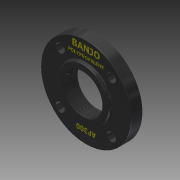
# Autodesk Inventor part: delta rythm
Saved by Autodesk Inventor 2013 SP2 (Build 170200200, 200)
## iProperties
Created: 2014-07-14
Part Number: delta rythm
Material: GFRP
Document SubType Name: Modeling
Designer: mrister
Density: 1.75 g/cm^3
Description: FLANGE, PLATIC - 3" 150#, THR'D (BANJO AF300)
Engineer: mrister
Author: mrister
Autodesk Inventor part; units mm, degrees
ref_plane "YZ Plane" through (0, 0, 0) normal (1, 0, 0) x (0, 1, 0)
ref_plane "XZ Plane" through (0, 0, 0) normal (0, 1, 0) x (-1, 0, 0)
ref_plane "XY Plane" through (0, 0, 0) normal (0, 0, 1) x (1, 0, 0)
sketch "Sketch1" plane through (0, 0, 0) normal (0, 0, 1) x (1, 0, 0)
  circle A0 centre (0, 0) radius 41.275
  circle A1 centre (0, 0) radius 95.25
  circle A2 centre (-53.8815, 53.8815) radius 9.525
  line L0 (-53.8815, 53.8815) -> (0, 0) construction
  line L1 (0, 0) -> (0, 95.25) construction
  circle A3 centre (-53.8815, -53.8815) radius 9.525
  circle A4 centre (53.8815, -53.8815) radius 9.525
  circle A5 centre (53.8815, 53.8815) radius 9.525
  dimension "d1" = 190.5
  dimension "d0" = 45
  dimension "d3" = 76.2
  dimension "d4" = 82.55
  dimension "d5" = 19.05
  dimension "d8" = 360
  constraints: 5 centre point, 4 end point, 2 coincident, 1 vertical, 1 vertical alignment, 11 other
  measures "d0" angle of L1 L0
  measures "d3" distance of L0.start L0.end
  measures "d4" diameter of A0
  measures "d5" diameter of A2
extrude "Extrusion1" add sketch "Sketch1" along normal blind 23.8125
sketch "Sketch2" plane through (0, 0, 23.8125) normal (0, 0, 1) x (1, 0, 0)
  circle A0 centre (0, 0) radius 41.275 projected
  circle A1 centre (0, 0) radius 95.25 projected
  circle A2 centre (0, 0) radius 53.975
  dimension "d12" = 107.95
  constraints: 1 centre point, 1 coincident
  measures "d12" diameter of A2
extrude "Extrusion2" add sketch "Sketch2" along normal blind 6.35 contours A2
chamfer "Chamfer1" distance 1.5875 angle 45 1 edges at (-53.975, 0, 23.8125)
fillet "Fillet1" radius 1.5875 2 edges at (-53.975, 0, 30.1625) (-95.25, 0, 23.8125)
sketch "Sketch3" plane through (0, 0, 0) normal (1, 0, 0) x (0, 1, 0)
  line L0 (41.275, 0) -> (41.275, 30.1625) projected
  line L1 (41.275, 35.0283) -> (41.275, 34.2346)
  line L2 (41.275, 34.2346) -> (42.0688, 34.6314)
  line L3 (42.0688, 34.6314) -> (41.275, 35.0283)
  line L4 (42.0688, 34.6314) -> (41.275, 34.6314) construction
  point P0 (0, 0)
  dimension "d20" = 0.7937
  constraints: 8 end point, 1 collinear, 1 horizontal, 1 midpoint, 1 perpendicular, 1 vertical
  measures "d20" distance of L1.start L1.end
coil "Coil1" sketch "Sketch3" operation cut axis through (0, 0, -10) along (0, 0, -1) pitch 0.9525 turns 160 hand right
sketch "Sketch4" plane through (0, 0, 23.8125) normal (0, 0, 1) x (1, 0, 0)
  circle A0 centre (0, 0) radius 93.6625 projected
  line L0 (-36.3748, 85.725) -> (36.3748, 85.725) construction
  line L1 (36.3748, 85.725) -> (36.3748, 60.325) construction
  line L2 (36.3748, 60.325) -> (-36.3748, 60.325) construction
  line L3 (-36.3748, 60.325) -> (-36.3748, 85.725) construction
  line L4 (0, 60.325) -> (0, 0) construction
  line L5 (12.7, -76.2) -> (-12.7, -76.2) construction
  line L6 (-12.7, -76.2) -> (-12.7, -63.5) construction
  line L7 (-12.7, -63.5) -> (12.7, -63.5) construction
  line L8 (12.7, -63.5) -> (12.7, -76.2) construction
  line L9 (0, -63.5) -> (0, 0) construction
  spline S0 degree 2 poles (-18.3296, 76.9511) (-18.3296, 76.0043) (-19.05, 74.5738) (-19.6469, 74.1003) knots 0 0 0 1 2 2 2
  spline S1 degree 2 poles (-19.6469, 74.1003) (-20.3673, 73.5343) (-22.0758, 73.0609) (-23.4034, 73.0609) knots 0 0 0 1 2 2 2
  line L10 (-23.4034, 73.0609) -> (-28.4772, 73.0609)
  line L11 (-28.4772, 73.0609) -> (-28.4772, 85.7609)
  line L12 (-28.4772, 85.7609) -> (-24.0003, 85.7609)
  spline S2 degree 2 poles (-24.0003, 85.7609) (-22.6006, 85.7609) (-21.1598, 85.5447) (-20.532, 85.2051) knots 0 0 0 1 2 2 2
  spline S3 degree 2 poles (-20.532, 85.2051) (-19.8425, 84.8449) (-19.1735, 83.6099) (-19.1735, 82.8071) knots 0 0 0 1 2 2 2
  spline S4 degree 2 poles (-19.1735, 82.8071) (-19.1735, 81.8809) (-20.0998, 80.4298) (-20.9231, 80.0901) knots 0 0 0 1 2 2 2
  line L13 (-20.9231, 80.0901) -> (-20.9231, 80.0284)
  spline S5 degree 2 poles (-20.9231, 80.0284) (-19.7395, 79.7814) (-18.3296, 78.2479) (-18.3296, 76.9511) knots 0 0 0 1 2 2 2
  spline S6 degree 2 poles (-21.6229, 77.0026) (-21.6229, 77.5995) (-22.0964, 78.2685) (-22.5698, 78.4435) knots 0 0 0 1 2 2 2
  spline S7 degree 2 poles (-22.5698, 78.4435) (-22.8579, 78.5567) (-23.8768, 78.5772) (-24.7207, 78.5772) knots 0 0 0 1 2 2 2
  line L14 (-24.7207, 78.5772) -> (-25.3074, 78.5772)
  line L15 (-25.3074, 78.5772) -> (-25.3074, 75.3765)
  line L16 (-25.3074, 75.3765) -> (-25.1324, 75.3765)
  spline S8 degree 2 poles (-25.1324, 75.3765) (-23.8974, 75.3765) (-22.9506, 75.4074) (-22.4566, 75.6235) knots 0 0 0 1 2 2 2
  spline S9 degree 2 poles (-22.4566, 75.6235) (-22.0243, 75.8191) (-21.6229, 76.5395) (-21.6229, 77.0026) knots 0 0 0 1 2 2 2
  spline S10 degree 2 poles (-22.4154, 82.1793) (-22.4154, 82.4881) (-22.7344, 83.1365) (-23.0638, 83.2806) knots 0 0 0 1 2 2 2
  spline S11 degree 2 poles (-23.0638, 83.2806) (-23.3725, 83.4246) (-24.237, 83.4452) (-25.0912, 83.4452) knots 0 0 0 1 2 2 2
  line L17 (-25.0912, 83.4452) -> (-25.3074, 83.4452)
  line L18 (-25.3074, 83.4452) -> (-25.3074, 80.7488)
  line L19 (-25.3074, 80.7488) -> (-24.906, 80.7488)
  spline S12 degree 2 poles (-24.906, 80.7488) (-24.0929, 80.7488) (-23.4343, 80.7797) (-23.0844, 80.9443) knots 0 0 0 1 2 2 2
  spline S13 degree 2 poles (-23.0844, 80.9443) (-22.7036, 81.1296) (-22.4154, 81.7574) (-22.4154, 82.1793) knots 0 0 0 1 2 2 2
  line L20 (-17.8664, 73.0609) -> (-13.5748, 85.7609)
  line L21 (-13.5748, 85.7609) -> (-10.0962, 85.7609)
  line L22 (-10.0962, 85.7609) -> (-5.8045, 73.0609)
  line L23 (-5.8045, 73.0609) -> (-9.0876, 73.0609)
  line L24 (-9.0876, 73.0609) -> (-9.8801, 75.6544)
  line L25 (-9.8801, 75.6544) -> (-13.8733, 75.6544)
  line L26 (-13.8733, 75.6544) -> (-14.676, 73.0609)
  line L27 (-14.676, 73.0609) -> (-17.8664, 73.0609)
  line L28 (-10.5799, 77.9597) -> (-11.8767, 82.1588)
  line L29 (-11.8767, 82.1588) -> (-13.1837, 77.9597)
  line L30 (-13.1837, 77.9597) -> (-10.5799, 77.9597)
  line L31 (6.3397, 73.0609) -> (3.2728, 73.0609)
  line L32 (3.2728, 73.0609) -> (-1.6261, 81.9118)
  line L33 (-1.6261, 81.9118) -> (-1.6261, 73.0609)
  line L34 (-1.6261, 73.0609) -> (-4.5387, 73.0609)
  line L35 (-4.5387, 73.0609) -> (-4.5387, 85.7609)
  line L36 (-4.5387, 85.7609) -> (-0.6278, 85.7609)
  line L37 (-0.6278, 85.7609) -> (3.4271, 78.4846)
  line L38 (3.4271, 78.4846) -> (3.4271, 85.7609)
  line L39 (3.4271, 85.7609) -> (6.3397, 85.7609)
  line L40 (6.3397, 85.7609) -> (6.3397, 73.0609)
  spline S14 degree 2 poles (15.1906, 76.7865) (15.1906, 75.9631) (14.6246, 74.5017) (14.0585, 73.9871) knots 0 0 0 1 2 2 2
  spline S15 degree 2 poles (14.0585, 73.9871) (13.4204, 73.4108) (11.6811, 72.8653) (10.549, 72.8653) knots 0 0 0 1 2 2 2
  spline S16 degree 2 poles (10.549, 72.8653) (9.7051, 72.8653) (8.2231, 72.9888) (7.6571, 73.1123) knots 0 0 0 1 2 2 2
  line L41 (7.6571, 73.1123) -> (7.6571, 75.6853)
  line L42 (7.6571, 75.6853) -> (7.9452, 75.6853)
  spline S17 degree 2 poles (7.9452, 75.6853) (8.326, 75.5309) (9.1596, 75.2633) (9.8183, 75.2633) knots 0 0 0 1 2 2 2
  spline S18 degree 2 poles (9.8183, 75.2633) (10.6622, 75.2633) (11.5782, 75.7367) (11.7635, 76.169) knots 0 0 0 1 2 2 2
  spline S19 degree 2 poles (11.7635, 76.169) (11.959, 76.5909) (12.0002, 77.6819) (12.0002, 78.3611) knots 0 0 0 1 2 2 2
  line L43 (12.0002, 78.3611) -> (12.0002, 83.4555)
  line L44 (12.0002, 83.4555) -> (9.0979, 83.4555)
  line L45 (9.0979, 83.4555) -> (9.0979, 85.7609)
  line L46 (9.0979, 85.7609) -> (15.1906, 85.7609)
  line L47 (15.1906, 85.7609) -> (15.1906, 76.7865)
  spline S20 degree 2 poles (29.2182, 79.4109) (29.2182, 76.3234) (25.9249, 72.7933) (23.0638, 72.7933) knots 0 0 0 1 2 2 2
  spline S21 degree 2 poles (23.0638, 72.7933) (20.1924, 72.7933) (16.9196, 76.3645) (16.9196, 79.4109) knots 0 0 0 1 2 2 2
  spline S22 degree 2 poles (16.9196, 79.4109) (16.9196, 82.4675) (20.1924, 86.0285) (23.0638, 86.0285) knots 0 0 0 1 2 2 2
  spline S23 degree 2 poles (23.0638, 86.0285) (25.9249, 86.0285) (29.2182, 82.4881) (29.2182, 79.4109) knots 0 0 0 1 2 2 2
  spline S24 degree 2 poles (25.9249, 79.4109) (25.9249, 80.5533) (25.4618, 82.1485) (25.0604, 82.6528) knots 0 0 0 1 2 2 2
  spline S25 degree 2 poles (25.0604, 82.6528) (24.659, 83.1776) (23.6298, 83.6305) (23.0741, 83.6305) knots 0 0 0 1 2 2 2
  spline S26 degree 2 poles (23.0741, 83.6305) (22.4874, 83.6305) (21.5303, 83.2085) (21.0878, 82.6734) knots 0 0 0 1 2 2 2
  spline S27 degree 2 poles (21.0878, 82.6734) (20.6967, 82.1793) (20.213, 80.543) (20.213, 79.4109) knots 0 0 0 1 2 2 2
  spline S28 degree 2 poles (20.213, 79.4109) (20.213, 78.2376) (20.6761, 76.6939) (21.0775, 76.169) knots 0 0 0 1 2 2 2
  spline S29 degree 2 poles (21.0775, 76.169) (21.4788, 75.6441) (22.5183, 75.1913) (23.0741, 75.1913) knots 0 0 0 1 2 2 2
  spline S30 degree 2 poles (23.0741, 75.1913) (23.6401, 75.1913) (24.6899, 75.675) (25.0707, 76.1896) knots 0 0 0 1 2 2 2
  spline S31 degree 2 poles (25.0707, 76.1896) (25.4823, 76.7453) (25.9249, 78.217) (25.9249, 79.4109) knots 0 0 0 1 2 2 2
  spline S32 degree 2 poles (-32.3083, 64.5036) (-32.3083, 64.061) (-32.5913, 63.2583) (-32.8538, 62.9907) knots 0 0 0 1 2 2 2
  spline S33 degree 2 poles (-32.8538, 62.9907) (-33.0133, 62.8209) (-33.4044, 62.543) (-33.636, 62.4452) knots 0 0 0 1 2 2 2
  spline S34 degree 2 poles (-33.636, 62.4452) (-33.8727, 62.3475) (-34.4233, 62.2343) (-34.7629, 62.2343) knots 0 0 0 1 2 2 2
  line L48 (-34.7629, 62.2343) -> (-35.5965, 62.2343)
  line L49 (-35.5965, 62.2343) -> (-35.5965, 60.1553)
  line L50 (-35.5965, 60.1553) -> (-37.1918, 60.1553)
  line L51 (-37.1918, 60.1553) -> (-37.1918, 66.5053)
  line L52 (-37.1918, 66.5053) -> (-34.7269, 66.5053)
  spline S35 degree 2 poles (-34.7269, 66.5053) (-34.1814, 66.5053) (-33.3838, 66.3046) (-33.0596, 66.0885) knots 0 0 0 1 2 2 2
  spline S36 degree 2 poles (-33.0596, 66.0885) (-32.6994, 65.8467) (-32.3083, 65.0542) (-32.3083, 64.5036) knots 0 0 0 1 2 2 2
  spline S37 degree 2 poles (-33.9447, 64.4624) (-33.9447, 64.7352) (-34.202, 65.1211) (-34.377, 65.1931) knots 0 0 0 1 2 2 2
  spline S38 degree 2 poles (-34.377, 65.1931) (-34.6034, 65.2909) (-35.0151, 65.3218) (-35.3701, 65.3218) knots 0 0 0 1 2 2 2
  line L53 (-35.3701, 65.3218) -> (-35.5965, 65.3218)
  line L54 (-35.5965, 65.3218) -> (-35.5965, 63.4178)
  line L55 (-35.5965, 63.4178) -> (-35.4833, 63.4178)
  spline S39 degree 2 poles (-35.4833, 63.4178) (-35.2621, 63.4178) (-34.8607, 63.4281) (-34.7114, 63.4538) knots 0 0 0 1 2 2 2
  spline S40 degree 2 poles (-34.7114, 63.4538) (-34.5828, 63.4744) (-34.2998, 63.5979) (-34.2226, 63.6751) knots 0 0 0 1 2 2 2
  spline S41 degree 2 poles (-34.2226, 63.6751) (-34.0579, 63.8295) (-33.9447, 64.1743) (-33.9447, 64.4624) knots 0 0 0 1 2 2 2
  spline S42 degree 2 poles (-25.6753, 63.3303) (-25.6753, 61.7866) (-27.322, 60.0215) (-28.7525, 60.0215) knots 0 0 0 1 2 2 2
  spline S43 degree 2 poles (-28.7525, 60.0215) (-30.1882, 60.0215) (-31.8246, 61.8072) (-31.8246, 63.3303) knots 0 0 0 1 2 2 2
  spline S44 degree 2 poles (-31.8246, 63.3303) (-31.8246, 64.8587) (-30.1882, 66.6391) (-28.7525, 66.6391) knots 0 0 0 1 2 2 2
  spline S45 degree 2 poles (-28.7525, 66.6391) (-27.322, 66.6391) (-25.6753, 64.8689) (-25.6753, 63.3303) knots 0 0 0 1 2 2 2
  spline S46 degree 2 poles (-27.322, 63.3303) (-27.322, 63.9015) (-27.5535, 64.6991) (-27.7542, 64.9513) knots 0 0 0 1 2 2 2
  spline S47 degree 2 poles (-27.7542, 64.9513) (-27.9549, 65.2137) (-28.4695, 65.4401) (-28.7474, 65.4401) knots 0 0 0 1 2 2 2
  spline S48 degree 2 poles (-28.7474, 65.4401) (-29.0407, 65.4401) (-29.5193, 65.2292) (-29.7405, 64.9616) knots 0 0 0 1 2 2 2
  spline S49 degree 2 poles (-29.7405, 64.9616) (-29.9361, 64.7146) (-30.1779, 63.8964) (-30.1779, 63.3303) knots 0 0 0 1 2 2 2
  spline S50 degree 2 poles (-30.1779, 63.3303) (-30.1779, 62.7437) (-29.9464, 61.9718) (-29.7457, 61.7094) knots 0 0 0 1 2 2 2
  spline S51 degree 2 poles (-29.7457, 61.7094) (-29.545, 61.4469) (-29.0253, 61.2205) (-28.7474, 61.2205) knots 0 0 0 1 2 2 2
  spline S52 degree 2 poles (-28.7474, 61.2205) (-28.4644, 61.2205) (-27.9395, 61.4624) (-27.7491, 61.7197) knots 0 0 0 1 2 2 2
  spline S53 degree 2 poles (-27.7491, 61.7197) (-27.5433, 61.9976) (-27.322, 62.7334) (-27.322, 63.3303) knots 0 0 0 1 2 2 2
  line L56 (-20.4934, 60.1553) -> (-24.7285, 60.1553)
  line L57 (-24.7285, 60.1553) -> (-24.7285, 66.5053)
  line L58 (-24.7285, 66.5053) -> (-23.1332, 66.5053)
  line L59 (-23.1332, 66.5053) -> (-23.1332, 61.3646)
  line L60 (-23.1332, 61.3646) -> (-20.4934, 61.3646)
  line L61 (-20.4934, 61.3646) -> (-20.4934, 60.1553)
  line L62 (-14.4522, 66.5053) -> (-16.6443, 62.8055)
  line L63 (-16.6443, 62.8055) -> (-16.6443, 60.1553)
  line L64 (-16.6443, 60.1553) -> (-18.2395, 60.1553)
  line L65 (-18.2395, 60.1553) -> (-18.2395, 62.7283)
  line L66 (-18.2395, 62.7283) -> (-20.4677, 66.5053)
  line L67 (-20.4677, 66.5053) -> (-18.6512, 66.5053)
  line L68 (-18.6512, 66.5053) -> (-17.411, 64.2412)
  line L69 (-17.411, 64.2412) -> (-16.2121, 66.5053)
  line L70 (-16.2121, 66.5053) -> (-14.4522, 66.5053)
  spline S54 degree 2 poles (-8.9924, 64.5036) (-8.9924, 64.061) (-9.2754, 63.2583) (-9.5379, 62.9907) knots 0 0 0 1 2 2 2
  spline S55 degree 2 poles (-9.5379, 62.9907) (-9.6974, 62.8209) (-10.0885, 62.543) (-10.32, 62.4452) knots 0 0 0 1 2 2 2
  spline S56 degree 2 poles (-10.32, 62.4452) (-10.5567, 62.3475) (-11.1074, 62.2343) (-11.447, 62.2343) knots 0 0 0 1 2 2 2
  line L71 (-11.447, 62.2343) -> (-12.2806, 62.2343)
  line L72 (-12.2806, 62.2343) -> (-12.2806, 60.1553)
  line L73 (-12.2806, 60.1553) -> (-13.8758, 60.1553)
  line L74 (-13.8758, 60.1553) -> (-13.8758, 66.5053)
  line L75 (-13.8758, 66.5053) -> (-11.411, 66.5053)
  spline S57 degree 2 poles (-11.411, 66.5053) (-10.8655, 66.5053) (-10.0679, 66.3046) (-9.7437, 66.0885) knots 0 0 0 1 2 2 2
  spline S58 degree 2 poles (-9.7437, 66.0885) (-9.3835, 65.8467) (-8.9924, 65.0542) (-8.9924, 64.5036) knots 0 0 0 1 2 2 2
  spline S59 degree 2 poles (-10.6288, 64.4624) (-10.6288, 64.7352) (-10.8861, 65.1211) (-11.061, 65.1931) knots 0 0 0 1 2 2 2
  spline S60 degree 2 poles (-11.061, 65.1931) (-11.2875, 65.2909) (-11.6991, 65.3218) (-12.0542, 65.3218) knots 0 0 0 1 2 2 2
  line L76 (-12.0542, 65.3218) -> (-12.2806, 65.3218)
  line L77 (-12.2806, 65.3218) -> (-12.2806, 63.4178)
  line L78 (-12.2806, 63.4178) -> (-12.1674, 63.4178)
  spline S61 degree 2 poles (-12.1674, 63.4178) (-11.9461, 63.4178) (-11.5448, 63.4281) (-11.3955, 63.4538) knots 0 0 0 1 2 2 2
  spline S62 degree 2 poles (-11.3955, 63.4538) (-11.2669, 63.4744) (-10.9839, 63.5979) (-10.9067, 63.6751) knots 0 0 0 1 2 2 2
  spline S63 degree 2 poles (-10.9067, 63.6751) (-10.742, 63.8295) (-10.6288, 64.1743) (-10.6288, 64.4624) knots 0 0 0 1 2 2 2
  line L79 (-2.2719, 60.1553) -> (-4.2119, 60.1553)
  line L80 (-4.2119, 60.1553) -> (-5.9769, 62.4864)
  line L81 (-5.9769, 62.4864) -> (-6.5533, 62.4864)
  line L82 (-6.5533, 62.4864) -> (-6.5533, 60.1553)
  line L83 (-6.5533, 60.1553) -> (-8.1382, 60.1553)
  line L84 (-8.1382, 60.1553) -> (-8.1382, 66.5053)
  line L85 (-8.1382, 66.5053) -> (-5.5858, 66.5053)
  spline S64 degree 2 poles (-5.5858, 66.5053) (-5.0558, 66.5053) (-4.2736, 66.3715) (-3.9392, 66.1657) knots 0 0 0 1 2 2 2
  spline S65 degree 2 poles (-3.9392, 66.1657) (-3.5995, 65.9496) (-3.1982, 65.2755) (-3.1982, 64.7609) knots 0 0 0 1 2 2 2
  spline S66 degree 2 poles (-3.1982, 64.7609) (-3.1982, 64.0353) (-3.8568, 63.1245) (-4.4074, 62.8569) knots 0 0 0 1 2 2 2
  line L86 (-4.4074, 62.8569) -> (-2.2719, 60.1553)
  spline S67 degree 2 poles (-4.8345, 64.5602) (-4.8345, 64.8021) (-5.0198, 65.1468) (-5.2308, 65.2395) knots 0 0 0 1 2 2 2
  spline S68 degree 2 poles (-5.2308, 65.2395) (-5.38, 65.3012) (-5.7454, 65.3372) (-6.0181, 65.3372) knots 0 0 0 1 2 2 2
  line L87 (-6.0181, 65.3372) -> (-6.5533, 65.3372)
  line L88 (-6.5533, 65.3372) -> (-6.5533, 63.6288)
  line L89 (-6.5533, 63.6288) -> (-6.0953, 63.6288)
  spline S69 degree 2 poles (-6.0953, 63.6288) (-5.7659, 63.6288) (-5.2977, 63.7111) (-5.1381, 63.8398) knots 0 0 0 1 2 2 2
  spline S70 degree 2 poles (-5.1381, 63.8398) (-4.9838, 63.9633) (-4.8345, 64.2926) (-4.8345, 64.5602) knots 0 0 0 1 2 2 2
  spline S71 degree 2 poles (3.9803, 63.3303) (3.9803, 61.7866) (2.3337, 60.0215) (0.9031, 60.0215) knots 0 0 0 1 2 2 2
  spline S72 degree 2 poles (0.9031, 60.0215) (-0.5326, 60.0215) (-2.169, 61.8072) (-2.169, 63.3303) knots 0 0 0 1 2 2 2
  spline S73 degree 2 poles (-2.169, 63.3303) (-2.169, 64.8587) (-0.5326, 66.6391) (0.9031, 66.6391) knots 0 0 0 1 2 2 2
  spline S74 degree 2 poles (0.9031, 66.6391) (2.3337, 66.6391) (3.9803, 64.8689) (3.9803, 63.3303) knots 0 0 0 1 2 2 2
  spline S75 degree 2 poles (2.3337, 63.3303) (2.3337, 63.9015) (2.1021, 64.6991) (1.9014, 64.9513) knots 0 0 0 1 2 2 2
  spline S76 degree 2 poles (1.9014, 64.9513) (1.7007, 65.2137) (1.1861, 65.4401) (0.9082, 65.4401) knots 0 0 0 1 2 2 2
  spline S77 degree 2 poles (0.9082, 65.4401) (0.6149, 65.4401) (0.1364, 65.2292) (-0.0849, 64.9616) knots 0 0 0 1 2 2 2
  spline S78 degree 2 poles (-0.0849, 64.9616) (-0.2804, 64.7146) (-0.5223, 63.8964) (-0.5223, 63.3303) knots 0 0 0 1 2 2 2
  spline S79 degree 2 poles (-0.5223, 63.3303) (-0.5223, 62.7437) (-0.2907, 61.9718) (-0.0901, 61.7094) knots 0 0 0 1 2 2 2
  spline S80 degree 2 poles (-0.0901, 61.7094) (0.1106, 61.4469) (0.6304, 61.2205) (0.9082, 61.2205) knots 0 0 0 1 2 2 2
  spline S81 degree 2 poles (0.9082, 61.2205) (1.1913, 61.2205) (1.7161, 61.4624) (1.9065, 61.7197) knots 0 0 0 1 2 2 2
  spline S82 degree 2 poles (1.9065, 61.7197) (2.1124, 61.9976) (2.3337, 62.7334) (2.3337, 63.3303) knots 0 0 0 1 2 2 2
  spline S83 degree 2 poles (9.8106, 64.5036) (9.8106, 64.061) (9.5276, 63.2583) (9.2651, 62.9907) knots 0 0 0 1 2 2 2
  spline S84 degree 2 poles (9.2651, 62.9907) (9.1056, 62.8209) (8.7145, 62.543) (8.483, 62.4452) knots 0 0 0 1 2 2 2
  spline S85 degree 2 poles (8.483, 62.4452) (8.2463, 62.3475) (7.6956, 62.2343) (7.356, 62.2343) knots 0 0 0 1 2 2 2
  line L90 (7.356, 62.2343) -> (6.5224, 62.2343)
  line L91 (6.5224, 62.2343) -> (6.5224, 60.1553)
  line L92 (6.5224, 60.1553) -> (4.9272, 60.1553)
  line L93 (4.9272, 60.1553) -> (4.9272, 66.5053)
  line L94 (4.9272, 66.5053) -> (7.392, 66.5053)
  spline S86 degree 2 poles (7.392, 66.5053) (7.9375, 66.5053) (8.7351, 66.3046) (9.0593, 66.0885) knots 0 0 0 1 2 2 2
  spline S87 degree 2 poles (9.0593, 66.0885) (9.4195, 65.8467) (9.8106, 65.0542) (9.8106, 64.5036) knots 0 0 0 1 2 2 2
  spline S88 degree 2 poles (8.1742, 64.4624) (8.1742, 64.7352) (7.9169, 65.1211) (7.742, 65.1931) knots 0 0 0 1 2 2 2
  spline S89 degree 2 poles (7.742, 65.1931) (7.5155, 65.2909) (7.1039, 65.3218) (6.7488, 65.3218) knots 0 0 0 1 2 2 2
  line L95 (6.7488, 65.3218) -> (6.5224, 65.3218)
  line L96 (6.5224, 65.3218) -> (6.5224, 63.4178)
  line L97 (6.5224, 63.4178) -> (6.6356, 63.4178)
  spline S90 degree 2 poles (6.6356, 63.4178) (6.8569, 63.4178) (7.2582, 63.4281) (7.4075, 63.4538) knots 0 0 0 1 2 2 2
  spline S91 degree 2 poles (7.4075, 63.4538) (7.5361, 63.4744) (7.8191, 63.5979) (7.8963, 63.6751) knots 0 0 0 1 2 2 2
  spline S92 degree 2 poles (7.8963, 63.6751) (8.061, 63.8295) (8.1742, 64.1743) (8.1742, 64.4624) knots 0 0 0 1 2 2 2
  line L98 (10.6648, 60.1553) -> (10.6648, 66.5053)
  line L99 (10.6648, 66.5053) -> (14.9565, 66.5053)
  line L100 (14.9565, 66.5053) -> (14.9565, 65.2961)
  line L101 (14.9565, 65.2961) -> (12.2497, 65.2961)
  line L102 (12.2497, 65.2961) -> (12.2497, 64.1794)
  line L103 (12.2497, 64.1794) -> (14.7455, 64.1794)
  line L104 (14.7455, 64.1794) -> (14.7455, 62.9701)
  line L105 (14.7455, 62.9701) -> (12.2497, 62.9701)
  line L106 (12.2497, 62.9701) -> (12.2497, 61.3646)
  line L107 (12.2497, 61.3646) -> (14.9565, 61.3646)
  line L108 (14.9565, 61.3646) -> (14.9565, 60.1553)
  line L109 (14.9565, 60.1553) -> (10.6648, 60.1553)
  line L110 (20.2721, 60.1553) -> (16.0371, 60.1553)
  line L111 (16.0371, 60.1553) -> (16.0371, 66.5053)
  line L112 (16.0371, 66.5053) -> (17.6323, 66.5053)
  line L113 (17.6323, 66.5053) -> (17.6323, 61.3646)
  line L114 (17.6323, 61.3646) -> (20.2721, 61.3646)
  line L115 (20.2721, 61.3646) -> (20.2721, 60.1553)
  line L116 (21.0337, 60.1553) -> (21.0337, 66.5053)
  line L117 (21.0337, 66.5053) -> (25.3254, 66.5053)
  line L118 (25.3254, 66.5053) -> (25.3254, 65.2961)
  line L119 (25.3254, 65.2961) -> (22.6187, 65.2961)
  line L120 (22.6187, 65.2961) -> (22.6187, 64.1794)
  line L121 (22.6187, 64.1794) -> (25.1144, 64.1794)
  line L122 (25.1144, 64.1794) -> (25.1144, 62.9701)
  line L123 (25.1144, 62.9701) -> (22.6187, 62.9701)
  line L124 (22.6187, 62.9701) -> (22.6187, 61.3646)
  line L125 (22.6187, 61.3646) -> (25.3254, 61.3646)
  line L126 (25.3254, 61.3646) -> (25.3254, 60.1553)
  line L127 (25.3254, 60.1553) -> (21.0337, 60.1553)
  line L128 (31.8452, 60.1553) -> (30.3117, 60.1553)
  line L129 (30.3117, 60.1553) -> (27.8623, 64.5808)
  line L130 (27.8623, 64.5808) -> (27.8623, 60.1553)
  line L131 (27.8623, 60.1553) -> (26.406, 60.1553)
  line L132 (26.406, 60.1553) -> (26.406, 66.5053)
  line L133 (26.406, 66.5053) -> (28.3614, 66.5053)
  line L134 (28.3614, 66.5053) -> (30.3889, 62.8672)
  line L135 (30.3889, 62.8672) -> (30.3889, 66.5053)
  line L136 (30.3889, 66.5053) -> (31.8452, 66.5053)
  line L137 (31.8452, 66.5053) -> (31.8452, 60.1553)
  line L138 (33.1368, 60.1553) -> (33.1368, 66.5053)
  line L139 (33.1368, 66.5053) -> (37.4285, 66.5053)
  line L140 (37.4285, 66.5053) -> (37.4285, 65.2961)
  line L141 (37.4285, 65.2961) -> (34.7217, 65.2961)
  line L142 (34.7217, 65.2961) -> (34.7217, 64.1794)
  line L143 (34.7217, 64.1794) -> (37.2175, 64.1794)
  line L144 (37.2175, 64.1794) -> (37.2175, 62.9701)
  line L145 (37.2175, 62.9701) -> (34.7217, 62.9701)
  line L146 (34.7217, 62.9701) -> (34.7217, 61.3646)
  line L147 (34.7217, 61.3646) -> (37.4285, 61.3646)
  line L148 (37.4285, 61.3646) -> (37.4285, 60.1553)
  line L149 (37.4285, 60.1553) -> (33.1368, 60.1553)
  line L150 (20.8446, -65.0875) -> (17.6259, -74.6125)
  line L151 (17.6259, -74.6125) -> (15.0169, -74.6125)
  line L152 (15.0169, -74.6125) -> (11.7982, -65.0875)
  line L153 (11.7982, -65.0875) -> (14.2605, -65.0875)
  line L154 (14.2605, -65.0875) -> (14.8548, -67.0326)
  line L155 (14.8548, -67.0326) -> (17.8497, -67.0326)
  line L156 (17.8497, -67.0326) -> (18.4518, -65.0875)
  line L157 (18.4518, -65.0875) -> (20.8446, -65.0875)
  line L158 (15.3797, -68.7616) -> (16.3523, -71.9109)
  line L159 (16.3523, -71.9109) -> (17.3326, -68.7616)
  line L160 (17.3326, -68.7616) -> (15.3797, -68.7616)
  line L161 (4.473, -72.7986) -> (8.4714, -72.7986)
  line L162 (8.4714, -72.7986) -> (8.4714, -71.0001)
  line L163 (8.4714, -71.0001) -> (4.7895, -71.0001)
  line L164 (4.7895, -71.0001) -> (4.7895, -69.1862)
  line L165 (4.7895, -69.1862) -> (8.4714, -69.1862)
  line L166 (8.4714, -69.1862) -> (8.4714, -65.0875)
  line L167 (8.4714, -65.0875) -> (10.8488, -65.0875)
  line L168 (10.8488, -65.0875) -> (10.8488, -74.6125)
  line L169 (10.8488, -74.6125) -> (4.473, -74.6125)
  line L170 (4.473, -74.6125) -> (4.473, -72.7986)
  spline S93 degree 2 poles (-3.5005, -67.9743) (-3.5005, -67.2719) (-2.9833, -66.1218) (-2.4816, -65.7204) knots 0 0 0 1 2 2 2
  spline S94 degree 2 poles (-2.4816, -65.7204) (-1.9799, -65.3191) (-0.6136, -64.8868) (0.3666, -64.8868) knots 0 0 0 1 2 2 2
  spline S95 degree 2 poles (0.3666, -64.8868) (1.4781, -64.8868) (3.0682, -65.2573) (3.5699, -65.4889) knots 0 0 0 1 2 2 2
  line L171 (3.5699, -65.4889) -> (3.5699, -67.5575)
  line L172 (3.5699, -67.5575) -> (3.3384, -67.5575)
  spline S96 degree 2 poles (3.3384, -67.5575) (2.8135, -67.2256) (1.401, -66.7316) (0.8143, -66.7316) knots 0 0 0 1 2 2 2
  spline S97 degree 2 poles (0.8143, -66.7316) (0.467, -66.7316) (-0.3435, -66.8551) (-0.6214, -67.0558) knots 0 0 0 1 2 2 2
  spline S98 degree 2 poles (-0.6214, -67.0558) (-0.8375, -67.2179) (-1.0999, -67.6887) (-1.0999, -68.1133) knots 0 0 0 1 2 2 2
  spline S99 degree 2 poles (-1.0999, -68.1133) (-1.0999, -68.5378) (-0.7294, -68.9932) (-0.4207, -69.1013) knots 0 0 0 1 2 2 2
  spline S100 degree 2 poles (-0.4207, -69.1013) (-0.1119, -69.2093) (0.7449, -69.2325) (1.0768, -69.2325) knots 0 0 0 1 2 2 2
  line L173 (1.0768, -69.2325) -> (1.4859, -69.2325)
  line L174 (1.4859, -69.2325) -> (1.4859, -70.9075)
  line L175 (1.4859, -70.9075) -> (1.1076, -70.9075)
  spline S101 degree 2 poles (1.1076, -70.9075) (0.6754, -70.9075) (-0.0579, -70.9847) (-0.3126, -71.1004) knots 0 0 0 1 2 2 2
  spline S102 degree 2 poles (-0.3126, -71.1004) (-0.5673, -71.2239) (-0.8529, -71.6562) (-0.8529, -72.0267) knots 0 0 0 1 2 2 2
  spline S103 degree 2 poles (-0.8529, -72.0267) (-0.8529, -72.32) (-0.5828, -72.6828) (-0.3898, -72.7831) knots 0 0 0 1 2 2 2
  spline S104 degree 2 poles (-0.3898, -72.7831) (-0.1582, -72.8989) (0.4593, -72.9761) (0.6754, -72.9761) knots 0 0 0 1 2 2 2
  spline S105 degree 2 poles (0.6754, -72.9761) (1.0227, -72.9761) (1.756, -72.814) (2.0957, -72.6828) knots 0 0 0 1 2 2 2
  spline S106 degree 2 poles (2.0957, -72.6828) (2.3658, -72.5825) (2.9524, -72.2583) (3.0914, -72.1734) knots 0 0 0 1 2 2 2
  line L176 (3.0914, -72.1734) -> (3.2921, -72.1734)
  line L177 (3.2921, -72.1734) -> (3.2921, -74.2111)
  spline S107 degree 2 poles (3.2921, -74.2111) (2.7981, -74.4195) (1.1308, -74.8132) (0.2586, -74.8132) knots 0 0 0 1 2 2 2
  spline S108 degree 2 poles (0.2586, -74.8132) (-0.5905, -74.8132) (-1.8409, -74.5199) (-2.2809, -74.2343) knots 0 0 0 1 2 2 2
  spline S109 degree 2 poles (-2.2809, -74.2343) (-2.7672, -73.9332) (-3.2535, -73.007) (-3.2535, -72.4281) knots 0 0 0 1 2 2 2
  spline S110 degree 2 poles (-3.2535, -72.4281) (-3.2535, -71.6099) (-2.3118, -70.3903) (-1.5399, -70.2128) knots 0 0 0 1 2 2 2
  line L178 (-1.5399, -70.2128) -> (-1.5399, -70.1202)
  spline S111 degree 2 poles (-1.5399, -70.1202) (-1.8795, -70.0738) (-2.5279, -69.8268) (-2.8367, -69.549) knots 0 0 0 1 2 2 2
  spline S112 degree 2 poles (-2.8367, -69.549) (-3.1223, -69.302) (-3.5005, -68.5146) (-3.5005, -67.9743) knots 0 0 0 1 2 2 2
  spline S113 degree 2 poles (-11.9603, -69.85) (-11.9603, -68.615) (-11.5666, -66.7625) (-11.1267, -66.1373) knots 0 0 0 1 2 2 2
  spline S114 degree 2 poles (-11.1267, -66.1373) (-10.6944, -65.5198) (-9.2973, -64.8868) (-8.2939, -64.8868) knots 0 0 0 1 2 2 2
  spline S115 degree 2 poles (-8.2939, -64.8868) (-7.2827, -64.8868) (-5.8933, -65.5198) (-5.4533, -66.1527) knots 0 0 0 1 2 2 2
  spline S116 degree 2 poles (-5.4533, -66.1527) (-5.0134, -66.7779) (-4.6197, -68.615) (-4.6197, -69.85) knots 0 0 0 1 2 2 2
  spline S117 degree 2 poles (-4.6197, -69.85) (-4.6197, -71.1159) (-5.0134, -72.9066) (-5.4611, -73.555) knots 0 0 0 1 2 2 2
  spline S118 degree 2 poles (-5.4611, -73.555) (-5.9087, -74.188) (-7.3213, -74.8055) (-8.2939, -74.8055) knots 0 0 0 1 2 2 2
  spline S119 degree 2 poles (-8.2939, -74.8055) (-9.3205, -74.8055) (-10.6944, -74.1571) (-11.1344, -73.5164) knots 0 0 0 1 2 2 2
  spline S120 degree 2 poles (-11.1344, -73.5164) (-11.5666, -72.8912) (-11.9603, -71.0464) (-11.9603, -69.85) knots 0 0 0 1 2 2 2
  spline S121 degree 2 poles (-9.5597, -69.85) (-9.5597, -71.6176) (-8.9808, -73.0456) (-8.2939, -73.0456) knots 0 0 0 1 2 2 2
  spline S122 degree 2 poles (-8.2939, -73.0456) (-7.6069, -73.0456) (-7.0202, -71.6176) (-7.0202, -69.8423) knots 0 0 0 1 2 2 2
  spline S123 degree 2 poles (-7.0202, -69.8423) (-7.0202, -68.0978) (-7.6069, -66.6467) (-8.2939, -66.6467) knots 0 0 0 1 2 2 2
  spline S124 degree 2 poles (-8.2939, -66.6467) (-8.9731, -66.6467) (-9.5597, -68.0978) (-9.5597, -69.85) knots 0 0 0 1 2 2 2
  spline S125 degree 2 poles (-20.3043, -69.85) (-20.3043, -68.615) (-19.9106, -66.7625) (-19.4707, -66.1373) knots 0 0 0 1 2 2 2
  spline S126 degree 2 poles (-19.4707, -66.1373) (-19.0384, -65.5198) (-17.6413, -64.8868) (-16.6379, -64.8868) knots 0 0 0 1 2 2 2
  spline S127 degree 2 poles (-16.6379, -64.8868) (-15.6267, -64.8868) (-14.2373, -65.5198) (-13.7974, -66.1527) knots 0 0 0 1 2 2 2
  spline S128 degree 2 poles (-13.7974, -66.1527) (-13.3574, -66.7779) (-12.9637, -68.615) (-12.9637, -69.85) knots 0 0 0 1 2 2 2
  spline S129 degree 2 poles (-12.9637, -69.85) (-12.9637, -71.1159) (-13.3574, -72.9066) (-13.8051, -73.555) knots 0 0 0 1 2 2 2
  spline S130 degree 2 poles (-13.8051, -73.555) (-14.2528, -74.188) (-15.6653, -74.8055) (-16.6379, -74.8055) knots 0 0 0 1 2 2 2
  spline S131 degree 2 poles (-16.6379, -74.8055) (-17.6645, -74.8055) (-19.0384, -74.1571) (-19.4784, -73.5164) knots 0 0 0 1 2 2 2
  spline S132 degree 2 poles (-19.4784, -73.5164) (-19.9106, -72.8912) (-20.3043, -71.0464) (-20.3043, -69.85) knots 0 0 0 1 2 2 2
  spline S133 degree 2 poles (-17.9038, -69.85) (-17.9038, -71.6176) (-17.3248, -73.0456) (-16.6379, -73.0456) knots 0 0 0 1 2 2 2
  spline S134 degree 2 poles (-16.6379, -73.0456) (-15.9509, -73.0456) (-15.3643, -71.6176) (-15.3643, -69.8423) knots 0 0 0 1 2 2 2
  spline S135 degree 2 poles (-15.3643, -69.8423) (-15.3643, -68.0978) (-15.9509, -66.6467) (-16.6379, -66.6467) knots 0 0 0 1 2 2 2
  spline S136 degree 2 poles (-16.6379, -66.6467) (-17.3171, -66.6467) (-17.9038, -68.0978) (-17.9038, -69.85) knots 0 0 0 1 2 2 2
  dimension "d30" = 25.4
  dimension "d32" = 60.325
  dimension "d33" = 25.4
  dimension "d34" = 12.7
  dimension "d35" = 63.5
  constraints: 4 end point, 2 midpoint, 2 vertical, 1 coincident, 1 parallel, 4 other
  measures "d30" distance of L2.end L0.start
  measures "d32" distance of L4.start L4.end
  measures "d33" distance of L5.start L5.end
  measures "d34" distance of L7.end L5.start
  measures "d35" distance of L9.start L4.end
extrude "Extrusion3" add sketch "Sketch4" along normal blind 0.0254 contours S0 S1 L10 L11 L12 S2 S3 S4 L13 S5 | L20 L21 L22 L23 L24 L25 L26 L27 | L31 L32 L33 L34 L35 L36 L37 L38 L39 L40 | S14 S15 S16 L41 L42 S17 S18 S19 L43 L44 L45 L46 L47 | S20 S21 S22 S23 | S32 S33 S34 L48 L49 L50 L51 L52 S35 S36 | S42 S43 S44 S45 | L56 L57 L58 L59 L60 L61 | L62 L63 L64 L65 L66 L67 L68 L69 L70 | S54 S55 S56 L71 L72 L73 L74 L75 S57 S58 | L79 L80 L81 L82 L83 L84 L85 S64 S65 S66 L86 | S71 S72 S73 S74 | S83 S84 S85 L90 L91 L92 L93 L94 S86 S87 | L98 L99 L100 L101 L102 L103 L104 L105 L106 L107 L108 L109 | L110 L111 L112 L113 L114 L115 | L116 L117 L118 L119 L120 L121 L122 L123 L124 L125 L126 L127 | L128 L129 L130 L131 L132 L133 L134 L135 L136 L137 | L138 L139 L140 L141 L142 L143 L144 L145 L146 L147 L148 L149 | L150 L151 L152 L153 L154 L155 L156 L157 | L161 L162 L163 L164 L165 L166 L167 L168 L169 L170 | S93 S94 S95 L171 L172 S96 S97 S98 S99 S100 L173 L174 L175 S101 S102 S103 S104 S105 S106 L176 L177 S107 S108 S109 S110 L178 S111 S112 | S113 S114 S115 S116 S117 S118 S119 S120 | S125 S126 S127 S128 S129 S130 S131 S132
body "Solid1"
